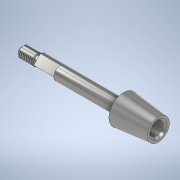
# Autodesk Inventor part: 2-阀门
Saved by Autodesk Inventor 2022 (Build 260153000, 153)
## iProperties
Created: 2023-01-24
Part Number: 2-阀门
Material: 不锈钢
Document SubType Name: Modeling
Designer: Lzy18
Density: 8 g/cm^3
Appearance: 半抛光
Author: Lzy18
Autodesk Inventor part; units mm, degrees
ref_plane "XZ Plane" through (0, 0, 0) normal (0, 1, 0) x (-1, 0, 0)
ref_plane "XY Plane" through (0, 0, 0) normal (0, 0, 1) x (1, 0, 0)
sketch "草图1" plane through (0, 0, 0) normal (0, 0, 1) x (1, 0, 0)
  line L0 (0, 0) -> (0, 4)
  line L1 (0, 4) -> (12, 4)
  line L2 (12, 4) -> (12, 3)
  line L3 (12, 3) -> (14, 3)
  line L4 (14, 3) -> (14, 5)
  line L5 (14, 5) -> (72.6225, 5)
  line L6 (72.6225, 5) -> (76, 10.85)
  line L7 (76, 10.85) -> (102, 8.25)
  line L8 (102, 8.25) -> (102, 0)
  line L9 (102, 0) -> (0, 0)
  dimension "d0" = 60
  dimension "d1" = 102
  dimension "d2" = 14
  dimension "d3" = 5
  dimension "d4" = 8.25
  dimension "d5" = 2
  dimension "d6" = 3
  dimension "d7" = 4
  dimension "d8" = 26
  dimension "d31" = 10.85
  dimension "d32" = 5.711
  constraints: 20 end point, 5 perpendicular, 2 vertical, 1 parallel
  measures "d0" angle of L9 L6
  measures "d1" distance between parallel lines of L0 L8
  measures "d2" distance between parallel lines of L0 L4
  measures "d3" distance between parallel lines of L9 L5
  measures "d4" distance from line of L7.end L9
  measures "d5" distance of L2.end L3.end
  measures "d6" distance between parallel lines of L9 L3
  measures "d7" distance between parallel lines of L9 L1
  measures "d8" distance from line of L8 L6.end
  measures "d31" distance from line of L9 L6.end
  measures "d32" angle of L9 L7
revolve "旋转1" add sketch "草图1" angle 360 about axis through (102, 0, 0) along (-1, 0, 0)
sketch "草图2" plane through (0, 0, 0) normal (0, 0, 1) x (1, 0, 0)
  line L0 (76, -10.85) -> (76, 10.85) projected
  line L1 (102, -8.25) -> (102, 8.25) projected
  line L2 (102, -8.25) -> (102, 8.25) projected
  line L3 (102, 0) -> (76, 0)
  line L4 (76, -10.85) -> (76, 10.85) projected
  circle A0 centre (86.5, 0) radius 5
  point P0 (0, 0)
  dimension "d10" = 10
  dimension "d11" = 15.5
  constraints: 2 end point, 2 midpoint, 1 centre point, 1 point on line
  measures "d10" diameter of A0
  measures "d11" distance from line of L1 A0.centre
extrude "拉伸1" cut sketch "草图2" against normal through all
sketch "草图3" plane through (0, 0, 0) normal (0, 0, 1) x (1, 0, 0)
  line L0 (76, -10.85) -> (76, 10.85) projected
  line L1 (102, -8.25) -> (102, 8.25) projected
  line L2 (102, -8.25) -> (102, 8.25) projected
  line L3 (102, -5) -> (80, -5)
  line L4 (80, -5) -> (76, 0)
  line L5 (76, 0) -> (102, 0)
  point P0 (0, 0)
  point P1 (86.7551, 4.9935)
  dimension "d14" = 5
  dimension "d15" = 22
  constraints: 6 end point, 2 midpoint, 1 perpendicular, 1 point on line, 1 other
  measures "d14" distance from line of L5 L3.start
  measures "d15" distance from line of L3.end L1
revolve "旋转2" cut sketch "草图3" angle 360 about axis through (76, 0, 0) along (1, 0, 0)
thread "螺纹1" size "M8x1.25" designation "M8" class "6g" standard "GB Metric profile" length 48
ref_plane "工作平面1" through (14, 0, 0) normal (1, 0, 0) x (0, 1, 0)
sketch "草图4" plane through (14, 0, 0) normal (1, 0, 0) x (0, 1, 0)
  circle A0 centre (0, 0) radius 5
  line L0 (0, 5) -> (-5, 0)
  circle A1 centre (0, 0) radius 5 projected
  line L1 (0, 5) -> (5, 0)
  point P0 (5, 0)
  dimension "d26" = 10
  constraints: 4 end point, 2 point on circle, 1 coincident, 1 perpendicular, 3 other
extrude "拉伸2" cut sketch "草图4" along normal blind 15 contours L1 A0 | L0 A0
chamfer "倒角3" distance 1.5 angle 45 2 edges at (0, -4, 0) (102, 5, 0)
